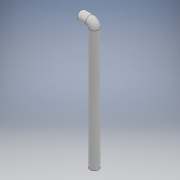
# Autodesk Inventor part: arm_stop
Saved by Autodesk Inventor 2018 (Build 220112000, 112)
## iProperties
Created: 2018-02-08
Part Number: arm_stop
Material: Generic
Document SubType Name: Modeling
Designer: suchanek
Density: 1 g/cm^3
Appearance: Default
Author: suchanek
Autodesk Inventor part; units mm, degrees
ref_plane "YZ Plane" through (0, 0, 0) normal (1, 0, 0) x (0, 1, 0)
ref_plane "XZ Plane" through (0, 0, 0) normal (0, 1, 0) x (-1, 0, 0)
ref_plane "XY Plane" through (0, 0, 0) normal (0, 0, 1) x (1, 0, 0)
sketch "Sketch1" plane through (0, 0, 0) normal (0, 0, 1) x (1, 0, 0)
  circle A0 centre (0, 0) radius 0.5
  dimension "d0" = 1
  constraints: 1 centre point, 1 coincident
  measures "d0" diameter of A0
sketch "Sketch2" plane through (0, 0, 0) normal (0, 1, 0) x (-1, 0, 0)
  line L0 (0.5, 15) -> (0.5, 15)
  line L1 (1.5, 14.5) -> (0.5, 14.5)
  line L2 (0, 0) -> (0, 14)
  arc A0 (0.5, 14.5) -> (0, 14) centre (0.5, 14) ccw
  dimension "d9" = 14
  dimension "d10" = 0.5
  dimension "d11" = 135
  dimension "d12" = 1
  constraints: 6 end point, 2 point on circle, 1 centre point, 1 vertical
  measures "d9" distance of L2.start L2.end
  measures "d10" radius of A0
  measures "d12" distance of L1.start L1.end
sweep "Sweep2" add profiles "Sketch1" path "Sketch2" path curves L2 A0 L1
body "Solid2"
